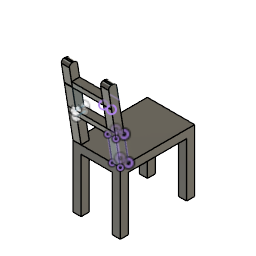
Record 9 (Autodesk Fusion 360 design; units mm, degrees)
Autodesk Fusion 360 part; units mm, degrees
sketch "Sketch1" plane through (0, 0, 0) normal (0, 1, 0) x (1, 0, 0)
  line L0 (0, 0) -> (-35, 0)
  line L1 (-35, 0) -> (-35, 6)
  line L2 (-35, 6) -> (0, 6)
  line L3 (0, 6) -> (0, 0)
  dimension "d3" = 35
  dimension "d4" = 6
  constraint horizontal L0
  constraint vertical L1
  constraint horizontal L2
  constraint vertical L3
  constraint coincident L0.start L3.end
  measures "d3" distance of L0.start L0.end
  measures "d4" distance of L0.start L2.end
extrude "Extrude1" add sketch "Sketch1" along normal blind 55
sketch "Sketch2" plane through (0, 0, -6) normal (0, 0, -1) x (1, 0, 0)
  line L0 (0, 0) -> (-35, 0)
  line L1 (-35, 0) -> (-35, -55)
  line L2 (-35, -55) -> (0, -55)
  line L3 (0, -55) -> (0, 0)
  line L4 (-35, 0) -> (-29, 0)
  line L5 (-29, 0) -> (-29, -6)
  line L6 (-29, -6) -> (-35, -6)
  line L7 (-35, -6) -> (-35, 0)
  line L8 (-6, -6) -> (-6, 0)
  line L9 (-6, 0) -> (0, 0)
  line L10 (0, -6) -> (-6, -6)
  line L11 (0, 0) -> (0, -6)
  line L12 (-35, -55) -> (-35, -49)
  line L13 (-35, -49) -> (-29, -49)
  line L14 (-29, -55) -> (-35, -55)
  line L15 (-29, -49) -> (-29, -55)
  line L16 (-6, -55) -> (-6, -49)
  line L17 (-6, -49) -> (0, -49)
  line L18 (0, -55) -> (-6, -55)
  line L19 (0, -49) -> (0, -55)
  dimension "d7" = 6
  dimension "d8" = 6
  dimension "d11" = 29
  dimension "d12" = -49
  constraint horizontal L4
  constraint vertical L5
  constraint horizontal L6
  constraint vertical L7
  constraint coincident L0.end L1.start
  measures "d7" distance of L0.end L4.end
  measures "d8" distance of L0.end L6.end
extrude "Extrude2" add sketch "Sketch2" along normal blind 40 contours L0 L3 L8 L9 L10 L11 | L0 L1 L4 L5 L6 L7 | L2 L3 L16 L17 L18 L19 | L1 L2 L12 L13 L14 L15
sketch "Sketch3" plane through (0, 0, 0) normal (1, 0, 0) x (0, 1, 0)
  line L0 (0, 0) -> (0, -46)
  line L1 (0, -46) -> (6, -46)
  line L2 (6, -46) -> (6, -6)
  line L3 (6, -6) -> (49, -6)
  line L4 (49, -6) -> (49, -46)
  line L5 (49, -46) -> (55, -46)
  line L6 (55, -46) -> (55, 0)
  line L7 (55, 0) -> (0, 0)
  line L8 (0, 0) -> (-9, 56)
  line L9 (-9, 56) -> (-3, 56)
  line L10 (-3, 56) -> (6, 0)
  dimension "d15" = 64
  dimension "d16" = 56
  dimension "d17" = 6
  constraint coincident L0.start L7.end
  constraint horizontal L9
  constraint coincident L7 L10.end
  constraint parallel L8 L10
  measures "d15" horizontal distance of L6.end L8.end
  measures "d16" vertical distance of L0.start L8.end
  measures "d17" distance of L8.end L9.end
extrude "Extrude3" add sketch "Sketch3" against normal blind 6 contours L7 L8 L9 L10
fillet "Fillet1" radius 3 1 edges at (-3, -3, 56)
fillet "Fillet1" radius 2 1 edges at (-3, -9, 56)
pattern_linear "R-Pattern1" count 2 spacing 29 along (-1, 0, 0) of "Extrude3"
fillet "Fillet2" radius 3 1 edges at (-32, -3, 56)
fillet "Fillet2" radius 2 1 edges at (-32, -9, 56)
sketch "Sketch4" plane through (0, 0, 0) normal (1, 0, 0) x (0, 1, 0)
  line L0 (-1.07, 44) -> (-7.0616, 44)
  line L1 (-0.4269, 40) -> (-6.4294, 40)
  line L2 (-7.0616, 44) -> (-7, 44)
  line L3 (-7.0616, 44) -> (-6.4294, 40)
  line L4 (-7.0616, 44) -> (-6.4294, 40)
  line L5 (-1.07, 44) -> (-0.4269, 40)
  line L6 (2.1496, 24) -> (-3.8609, 24)
  line L7 (-3.8609, 24) -> (-3.2233, 20)
  line L8 (-3.2233, 20) -> (2.7872, 20)
  line L9 (2.7872, 20) -> (2.1496, 24)
  point P0 (-6.6529, 56)
  dimension "d32" = 12
  dimension "d33" = 4
  dimension "d34" = 16
  dimension "d35" = 4
  constraint horizontal L0
  constraint parallel L0 L1
  constraint coincident L0 L2.end
  constraint coincident L1 L3.end
  constraint horizontal L6
  constraint horizontal L8
  constraint parallel L7 L9
  measures "d32" vertical distance of L0.end P0
  measures "d33" vertical distance of L0.end L1.end
  measures "d34" distance of L1 L6
  measures "d35" vertical distance of L6.end L7.end
extrude "Extrude4" add sketch "Sketch4" against normal blind 35
sketch "Sketch5" plane through (0, 0, 0) normal (0, -0.98733, -0.158678) x (1, 0, 0)
  line L0 (0, 54.3715) -> (-6, 54.3715)
  line L1 (-6, 54.3715) -> (-6, 40.8346)
  line L2 (-6, 0) -> (0, 0)
  line L3 (0, 40.8346) -> (0, 54.3715)
  line L4 (0, 20.2566) -> (-6, 20.2566)
  line L5 (-6, 20.2566) -> (-6, 0)
  line L6 (0, 0) -> (0, 20.2566)
sketch "Sketch6" plane through (0, 5.8489, 0.94) normal (0, 0.98733, 0.158678) x (-1, 0, 0)
  line L0 (6, 53.2102) -> (0, 53.2102)
  line L1 (0, 53.2102) -> (0, 43.6125)
  line L2 (0, -0.9521) -> (6, -0.9521)
  line L3 (6, 43.6125) -> (6, 53.2102)
  line L4 (0, 43.6125) -> (6, 43.6125)
  line L5 (6, 19.3046) -> (0, 19.3046)
  line L6 (0, 19.3046) -> (0, -0.9521)
  line L7 (6, -0.9521) -> (6, 19.3046)
sketch "Sketch7" plane through (-29, 0, 0) normal (1, 0, 0) x (0, 1, 0)
  line L0 (-0.4286, 40) -> (-6.4286, 40)
  line L1 (-6.4286, 40) -> (-3.8571, 24)
  line L2 (-3.8571, 24) -> (2.1429, 24)
  line L3 (2.1429, 24) -> (-0.4286, 40)
  line L4 (-3.2504, 20.0179) -> (2.8037, 20.0179)
  line L5 (-3.8548, 23.9842) -> (2.1102, 23.9842)
  constraint horizontal L4
  constraint parallel L2 L5
